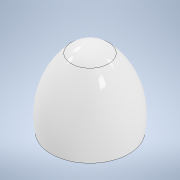
# Autodesk Inventor part: SmartEgg Shell Top
Saved by Autodesk Inventor 2020 (Build 240168000, 168)
## iProperties
Created: 2019-11-26
Part Number: SmartEgg Shell Top
Material: Generic
Document SubType Name: Modeling
Designer: Andrew
Density: 1 g/cm^3
Appearance: White
Author: Andrew
Autodesk Inventor part; units mm, degrees
ref_plane "YZ Plane" through (0, 0, 0) normal (1, 0, 0) x (0, 1, 0)
ref_plane "XZ Plane" through (0, 0, 0) normal (0, 1, 0) x (-1, 0, 0)
ref_plane "XY Plane" through (0, 0, 0) normal (0, 0, 1) x (1, 0, 0)
derived "SmartEgg Shell.ipt"
sketch "Shell Sketch" plane through (0, -10.3291, -13.7529) normal (0, 0.792624, -0.6097108) x (0, 0.6097108, 0.792624)
  arc A0 (40.9669, -18.122) -> (29.5168, 33.2086) centre (-6.2647, -1.7154) ccw
  arc A1 (17.3511, -34.9187) -> (29.8511, -31.5693) centre (17.3511, -9.9187) ccw construction
  line L0 (17.3511, -34.9187) -> (17.3511, -31.5693) construction
  line L1 (17.3511, 9.75) -> (36.2021, 9.75)
  line L2 (17.3511, 26.5) -> (17.3511, -26.5) construction
  line L3 (34.7021, -26.5) -> (35.4251, -27.1909) construction
  arc A2 (29.5168, 33.2086) -> (17.3511, 38.3345) centre (17.3511, 21.3345) ccw
  line L4 (17.3511, 38.3345) -> (17.3511, 35.4766)
  line L5 (17.3511, 35.4766) -> (22.3511, 35.4766)
  arc A3 (28.0855, 31.8117) -> (22.3511, 35.4766) centre (17.3511, 21.3345) ccw
  arc A4 (37.2672, 18.5076) -> (28.0855, 31.8117) centre (-6.2647, -1.7154) ccw
  arc A5 (34.7021, 22) -> (30.2021, 26.5) centre (30.2021, 22) ccw construction
  line L6 (36.2021, 9.75) -> (36.2021, -11.5693)
  line L7 (36.2021, -11.5693) -> (42.7547, -11.5693)
  line L8 (39.2021, 9.75) -> (39.2021, -11.3193)
  line L9 (39.2021, -11.3193) -> (42.8042, -11.3193)
  line L10 (17.3511, -31.5693) -> (29.8511, -31.5693)
  arc A6 (29.8511, -31.5693) -> (40.9669, -18.122) centre (17.3511, -9.9187) ccw
  line L11 (17.3511, -31.5693) -> (17.3511, 9.75)
  line L12 (34.7021, -26.5) -> (34.7021, 22) construction
  line L13 (20.552, 10.75) -> (17.1986, 10.75) construction
  arc A7 (39.2021, 9.75) -> (37.2672, 18.5076) centre (18.4156, 9.75) ccw
  point P0 (17.1986, 0)
  point P1 (39.2021, 13.6718)
sketch "Thread Sketch" plane through (0, -10.3291, -13.7529) normal (0, 0.792624, -0.6097108) x (0, 0.6097108, 0.792624)
  line L0 (36.2021, 9.75) -> (36.2021, -11.5693) construction
  line L1 (39.2021, 9.75) -> (39.2021, -11.3193) construction
  line L2 (36.2021, 9.75) -> (38.7021, 7.25)
  line L3 (38.7021, 7.25) -> (38.7021, 5.25)
  line L4 (38.7021, 5.25) -> (36.2021, 2.75)
  line L5 (36.2021, 2.75) -> (36.2021, 9.75)
  line L6 (39.2021, 5.3964) -> (36.7021, 2.8964)
  line L7 (36.7021, 2.8964) -> (36.7021, 0.8964)
  line L8 (36.7021, 0.8964) -> (39.2021, -1.6036)
  line L9 (39.2021, -1.6036) -> (39.2021, 5.3964)
  line L10 (38.7021, 6.25) -> (36.2021, 6.25) construction
  line L11 (36.7021, 1.8964) -> (39.2021, 1.8964) construction
  point P0 (17.1986, 0)
sketch "Thread Mask" plane through (0, -10.3291, -13.7529) normal (0, 0.792624, -0.6097108) x (0, 0.6097108, 0.792624)
  line L0 (39.2021, 7.25) -> (36.2021, 7.25)
  line L1 (36.2021, 7.25) -> (36.2021, -11.5693)
  line L2 (36.2021, -11.5693) -> (39.2021, -11.5693)
  line L3 (39.2021, -11.5693) -> (39.2021, 7.25)
  line L4 (36.2021, 9.75) -> (36.2021, -11.5693) construction
  line L5 (39.2021, 9.75) -> (39.2021, -11.3193) construction
  point P0 (17.1986, 0)
revolve "Revolution1" add sketch "Shell Sketch" angle 360 about axis through (-31.5693, 0.25, 0) along (1, 0, 0) contours L9 L8 A7 A4 A3 L5 L4 A2 A0
coil "Coil1" sketch "Thread Sketch" operation add axis through (-31.5693, 0.25, 0) along (-1, 0, 0) pitch 8.708 turns 3 hand right separate body contours L9 L8 L7 L6
coil "Coil2" sketch "Thread Sketch" operation add axis through (-31.5693, 0.25, 0) along (1, 0, 0) pitch 8.708 turns 3 hand right bodies 2 contours L9 L8 L7 L6
sketch "Top Thread Mask" plane through (0, -10.3291, -13.7529) normal (0, 0.792624, -0.6097108) x (0, 0.6097108, 0.792624)
  arc A0 (39.2021, 9.75) -> (37.2672, 18.5076) centre (18.4156, 9.75) ccw projected
  arc A1 (37.2672, 18.5076) -> (28.0855, 31.8117) centre (-6.2647, -1.7154) ccw projected
  arc A2 (28.0855, 31.8117) -> (22.3511, 35.4766) centre (17.3511, 21.3345) ccw projected
  line L0 (17.3511, 35.4766) -> (22.3511, 35.4766) projected
  line L1 (17.3511, 35.4766) -> (17.3511, -11.3193)
  line L2 (17.3511, -11.3193) -> (39.2021, -11.3193)
  line L3 (39.2021, -11.3193) -> (39.2021, 9.75)
  line L4 (39.2021, -11.3193) -> (42.8042, -11.3193) construction
  point P0 (17.1986, 0)
  constraints: 6 end point, 2 vertical, 1 collinear, 1 perpendicular
revolve "Revolution2" cut sketch "Top Thread Mask" angle 360 about axis through (35.4766, 0.25, 0) along (-1, 0, 0) keep common part bodies 2
combine bodies "Combine1" operation type add bodies to combine 1 2
ref_plane "Work Plane2" through (0, -10.3291, -13.7529) normal (0, 0.792624, -0.6097108) x (0, 0.6097108, 0.792624)
equation "\"d2\" = 2 * Thread_Pitch"
equation "\"d10\" = 2 * Thread_Pitch"
equation "\"Thread_Pitch\" = 4.354"
body "Solid1"
